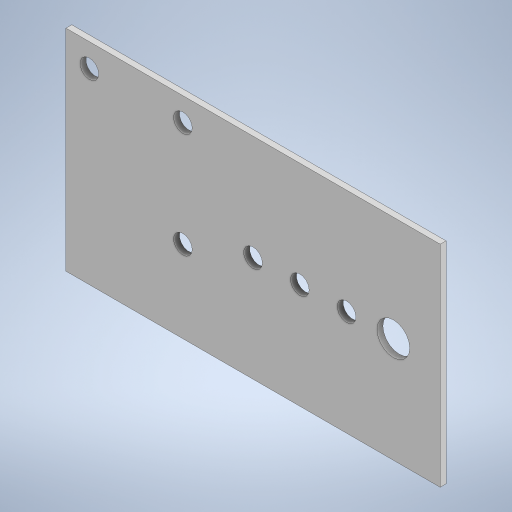
# Autodesk Inventor part: flatPoly2ForCNC
Saved by Autodesk Inventor 2023.4 (Build 274418000, 418)
## iProperties
Created: 2023-12-19
Part Number: flatPoly2ForCNC
Material: Generic
Document SubType Name: Modeling
Designer: Meer
Density: 1 g/cm^3
Appearance: Default
Author: Meer
Autodesk Inventor part; units mm, degrees
ref_plane "YZ Plane" through (0, 0, 0) normal (1, 0, 0) x (0, 1, 0)
ref_plane "XZ Plane" through (0, 0, 0) normal (0, 1, 0) x (-1, 0, 0)
ref_plane "XY Plane" through (0, 0, 0) normal (0, 0, 1) x (1, 0, 0)
sketch "Sketch1" plane through (0, 0, 0) normal (0, 0, 1) x (1, 0, 0)
  line L0 (0, 0) -> (101.6, 0)
  line L1 (101.6, 0) -> (101.6, 57.15)
  line L2 (101.6, 57.15) -> (0, 57.15)
  line L3 (0, 57.15) -> (0, 0)
  line L4 (2.6205, 15.875) -> (101.6, 15.875)
  line L5 (2.6205, 15.875) -> (0, 15.875)
  circle A0 centre (88.9, 28.575) radius 4.445
  circle A1 centre (76.2, 28.575) radius 2.54
  circle A2 centre (63.5, 28.575) radius 2.54
  circle A3 centre (50.8, 28.575) radius 2.54
  circle A4 centre (31.75, 22.225) radius 2.54
  circle A5 centre (6.35, 50.8) radius 2.54
  circle A6 centre (31.75, 50.8) radius 2.54
  dimension "d0" = 101.6
  dimension "d1" = 57.15
  dimension "d7" = 8.89
  dimension "d11" = 5.08
  dimension "d12" = 5.08
  dimension "d13" = 5.08
  dimension "d16" = 5.08
  dimension "d21" = 5.08
  dimension "d23" = 5.08
  constraints: 12 end point, 7 centre point, 3 perpendicular, 2 parallel, 2 point on line, 1 horizontal
  measures "d0" distance of L1.end L2.end
  measures "d1" distance of L0.end L1.end
  measures "d7" diameter of A0
  measures "d11" diameter of A1
  measures "d12" diameter of A2
  measures "d13" diameter of A3
  measures "d16" diameter of A4
  measures "d21" diameter of A5
  measures "d23" diameter of A6
extrude "Extrusion2" add sketch "Sketch1" along normal blind 1.5875
body "Solid2"
